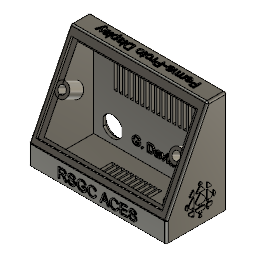
HalfSizeDisplayv4 (Autodesk Fusion 360 design; units mm, degrees)
Autodesk Fusion 360 part; units mm, degrees
sketch "Base" plane through (0, 0, 0) normal (0, 0, 1) x (1, 0, 0)
  line L0 (44.45, -19.685) -> (-44.45, -19.685)
  line L1 (-44.45, -19.685) -> (-44.45, 19.685)
  line L2 (-44.45, 19.685) -> (44.45, 19.685)
  line L3 (44.45, 19.685) -> (44.45, -19.685)
  line L4 (44.45, -19.685) -> (-44.45, 19.685) construction
  line L5 (-44.45, -19.685) -> (44.45, 19.685) construction
  line L6 (38.1, 15.875) -> (-38.1, 15.875)
  line L7 (-38.1, 15.875) -> (-38.1, -15.875)
  line L8 (-38.1, -15.875) -> (38.1, -15.875)
  line L9 (38.1, -15.875) -> (38.1, 15.875)
  line L10 (38.1, 15.875) -> (-38.1, -15.875) construction
  line L11 (-38.1, 15.875) -> (38.1, -15.875) construction
  dimension "d1" = 88.9
  dimension "d2" = 39.37
  dimension "d30" = 76.2
  dimension "d31" = 31.75
  constraint horizontal L0
  constraint perpendicular L0 L1
  constraint parallel L0 L2
  constraint parallel L1 L3
  constraint coincident L4 origin
  constraint coincident L5 origin
  constraint horizontal L6
  constraint perpendicular L6 L7
  constraint parallel L6 L8
  constraint parallel L7 L9
  constraint coincident L10 origin
  constraint coincident L11 origin
  measures "d1" distance of L1.end L2.end
  measures "d2" distance of L0.end L1.end
  measures "d30" distance of L7.end L8.end
  measures "d31" distance of L6.end L7.end
extrude "Extrude1" add sketch "Base" along normal blind 66.04 contours L0 L1 L2 L3 | L6 L7 L8 L9 makes body 1
sketch "2Points" plane through (44.45, 0, 0) normal (1, 0, 0) x (0, 1, 0)
  line L0 (-19.685, 0) -> (19.685, 0)
  line L1 (19.685, 0) -> (19.685, 66.04)
  line L2 (19.685, 66.04) -> (-19.685, 66.04)
  line L3 (-19.685, 66.04) -> (-19.685, 0)
  line L4 (6.9804, 66.04) -> (-19.685, 12.7041)
  point P0 (6.9804, 66.04)
  point P1 (-19.685, 12.7041)
  constraint coincident L2 P0
  constraint coincident L3 P1
  constraint coincident P0 L4.start
  constraint coincident P1 L4.end
sketch "BaseFill" plane through (0, 0, 0) normal (0, 0, -1) x (1, 0, 0)
  line L0 (-44.45, -19.685) -> (44.45, -19.685)
  line L1 (44.45, -19.685) -> (44.45, 19.685)
  line L2 (44.45, 19.685) -> (-44.45, 19.685)
  line L3 (-44.45, 19.685) -> (-44.45, -19.685)
  line L4 (-39.37, 14.605) -> (-39.37, -14.605)
  line L5 (-39.37, -14.605) -> (39.37, -14.605)
  line L6 (39.37, -14.605) -> (39.37, 14.605)
  line L7 (39.37, 14.605) -> (-39.37, 14.605)
  dimension "d5" = -5.08
extrude "Extrude3" cut sketch "2Points" against normal blind 101.6 contours L2 L3 L4 bodies 1
sketch "PermaProto" plane through (0, -20.83, 10.414) normal (0, -0.894444, 0.44718) x (1, 0, 0)
  line L0 (-44.45, 62.1906) -> (-44.45, 2.5604)
  line L1 (-44.45, 2.5604) -> (44.45, 2.5604)
  line L2 (44.45, 2.5604) -> (44.45, 62.1906)
  line L3 (44.45, 62.1906) -> (-44.45, 62.1906)
  line L4 (40.259, 57.023) -> (-41.275, 57.023)
  line L5 (-41.275, 57.023) -> (-41.275, 5.969)
  line L6 (-41.275, 5.969) -> (40.259, 5.969)
  line L7 (40.259, 5.969) -> (40.259, 57.023)
  line L8 (40.259, 57.023) -> (-41.275, 5.969) construction
  line L9 (-41.275, 57.023) -> (40.259, 5.969) construction
  point P0 (-0.508, 31.496)
  dimension "d25" = 81.534
  dimension "d26" = 51.054
  constraint horizontal L4
  constraint perpendicular L4 L5
  constraint parallel L4 L6
  constraint parallel L5 L7
  constraint coincident L8 P0
  constraint coincident L9 P0
  measures "d25" distance of L5.end L6.end
  measures "d26" distance of L4.end L5.end
extrude "Extrude6" cut sketch "PermaProto" against normal blind 1.5748 contours L4 L5 L6 L7 bodies 1
extrude "Extrude7" cut sketch "Base" along normal blind 59.69 contours L6 L7 L8 L9 bodies 1
fillet "Fillet5" radius 1.27 1 edges at (44.45, -19.685, 6.3521) on bodies 1
fillet "Fillet6" radius 1.27 1 edges at (-44.45, -19.685, 6.3521) on bodies 1
sketch "RSGC ACES" plane through (0, -19.685, 0) normal (0, -1, 0) x (1, 0, 0)
  line L0 (-43.18, 12.7041) -> (-43.18, 0)
  line L1 (-43.18, 0) -> (43.18, 0)
  line L2 (43.18, 0) -> (43.18, 12.7041)
  line L3 (43.18, 12.7041) -> (-43.18, 12.7041)
  line L4 (-35.052, 1.524) -> (35.56, 1.524) construction
  line L5 (35.56, 1.524) -> (35.56, 10.16) construction
  line L6 (35.56, 10.16) -> (-35.052, 10.16) construction
  line L7 (-35.052, 10.16) -> (-35.052, 1.524) construction
  dimension "d38" = 6.35
  text T0 "RSGC ACES" font "Arial" height 6.35 align centre middle in box 70.612 x 8.636 at (-35.052, 1.524) x (1, 0) y (0, 1) spacing 1 kerned
extrude "Extrude8" add sketch "RSGC ACES" along normal blind 0.508 text T0 bodies 1
fillet "Fillet7" radius 1.27 1 edges at (44.45, 19.685, 33.02) on bodies 1
fillet "Fillet8" radius 1.27 1 edges at (-44.45, 19.685, 33.02) on bodies 1
sketch "TopText" plane through (0, 0, 66.04) normal (0, 0, 1) x (-1, 0, 0)
  arc A0 (43.18, -19.685) -> (44.45, -18.415) centre (43.18, -18.415) ccw
  line L0 (44.45, -18.415) -> (44.45, -6.9804)
  line L1 (44.45, -6.9804) -> (-44.45, -6.9804)
  line L2 (-44.45, -6.9804) -> (-44.45, -18.415)
  arc A1 (-44.45, -18.415) -> (-43.18, -19.685) centre (-43.18, -18.415) ccw
  line L3 (-43.18, -19.685) -> (43.18, -19.685)
  line L4 (-44.2048, -20.7361) -> (45.0445, -20.5016) construction
  line L5 (45.0445, -20.5016) -> (45.0031, -4.76) construction
  line L6 (45.0031, -4.76) -> (-44.2462, -4.9945) construction
  line L7 (-44.2462, -4.9945) -> (-44.2048, -20.7361) construction
  dimension "d45" = 5.08
  text T0 "Perma-Proto Display" font "Arial" height 5.08 align centre middle in box 89.2496 x 15.7417 at (-44.2048, -20.7361) x (0.999997, 0.002627) y (-0.002627, 0.999997) spacing 1 kerned
extrude "Extrude9" add sketch "TopText" along normal blind 0.508 text T0 bodies 1
fillet "Fillet9" radius 1.27 5 edges at (44.45, -5.7173, 40.6422) (44.078, -19.313, 13.4481) (0, -19.685, 12.7041) (-44.078, -19.313, 13.4481) (-44.45, -5.7173, 40.6422) on bodies 1
fillet "Fillet10" radius 1.27 8 edges at (44.078, 7.3963, 66.04) (44.45, 13.4077, 66.04) (44.078, 19.313, 66.04) (0, 19.685, 66.04) (-44.078, 19.313, 66.04) (-44.45, 13.4077, 66.04) (-44.078, 7.3963, 66.04) (0, 6.9804, 66.04) on bodies 1
sketch "Revised_ACESLogoOutline-01" plane through (44.45, 0, 0) normal (1, 0, 0) x (0, 1, 0)
  arc A0 (1.4641, 12.3032) -> (0.4552, 12.1444) centre (0.401, 15.7741) cw
  spline S0 degree 3 poles (0.4552, 12.1444) (-0.3472, 12.1908) (-1.0048, 12.7982) (-1.1147, 13.5944) knots 1 1 1 1 2 2 2 2
  arc A1 (-1.1147, 13.5944) -> (-0.6596, 14.9843) centre (0.7846, 13.742) cw
  spline S1 degree 3 poles (-0.6596, 14.9843) (0.0742, 15.8839) (0.8185, 16.7764) (1.5523, 17.6795) knots 3 3 3 3 4 4 4 4
  spline S2 degree 3 poles (1.5523, 17.6795) (1.7123, 17.8877) (2.0105, 17.9271) (2.219, 17.7677) knots 4 4 4 4 5 5 5 5
  arc A2 (2.219, 17.7677) -> (2.3072, 17.6795) centre (1.9721, 17.4326) cw
  spline S3 degree 3 poles (2.3072, 17.6795) (2.7482, 17.1186) (3.2174, 16.5859) (3.669, 16.0356) knots 6 6 6 6 7 7 7 7
  arc A3 (3.669, 16.0356) -> (4.685, 14.7726) centre (-6.6786, 6.6712) cw
  spline S4 degree 3 poles (4.685, 14.7726) (5.2142, 14.0329) (5.0455, 13.0043) (4.3075, 12.4725) knots 8 8 8 8 9 9 9 9
  arc A4 (4.3075, 12.4725) -> (3.7219, 12.2079) centre (3.3301, 13.8553) cw
  arc A5 (3.7219, 12.2079) -> (2.5895, 12.2644) centre (3.2701, 14.5316) cw
  spline S5 degree 3 poles (2.5895, 12.2644) (2.526, 12.2644) (2.4413, 12.3455) (2.3566, 12.2397) (2.4237, 12.1656) (2.4448, 12.1021) knots 11 11 11 11 12 12 13 13 13 13
  arc A6 (2.4448, 12.1021) -> (2.8082, 11.4565) centre (6.0267, 13.6931) ccw
  spline S6 degree 3 poles (2.8082, 11.4565) (2.854, 11.386) (2.914, 11.3119) (2.8082, 11.1284) (2.72, 11.1461) (2.6318, 11.1461) knots 14 14 14 14 15 15 16 16 16 16
  line L0 (2.6318, 11.1461) -> (1.2207, 11.1461)
  arc A7 (1.2207, 11.1461) -> (1.0408, 11.2272) centre (1.2028, 11.3464) cw
  spline S7 degree 3 poles (1.0408, 11.2272) (0.9914, 11.3013) (1.0408, 11.3613) (1.069, 11.4213) knots 18 18 18 18 19 19 19 19
  arc A8 (1.069, 11.4213) -> (1.4641, 12.3032) centre (-1.2514, 12.9903) ccw
  arc A9 (2.3813, 8.1581) -> (2.7694, 7.3008) centre (5.1756, 8.9065) ccw
  arc A10 (2.7694, 7.3008) -> (2.8364, 7.202) centre (2.0017, 6.7077) cw
  spline S8 degree 3 poles (2.8364, 7.202) (2.8778, 7.1337) (2.856, 7.0448) (2.7876, 7.0034) knots 2 2 2 2 3 3 3 3
  spline S9 degree 3 poles (2.7876, 7.0034) (2.7863, 7.0025) (2.7849, 7.0017) (2.7835, 7.0009) knots 3 3 3 3 4 4 4 4
  arc A11 (2.7835, 7.0009) -> (2.6988, 6.9798) centre (2.7131, 7.1024) cw
  line L1 (2.6988, 6.9798) -> (1.1501, 6.9798)
  spline S10 degree 3 poles (1.1501, 6.9798) (1.0055, 6.9798) (0.949, 7.0927) (1.0267, 7.2197) knots 6 6 6 6 7 7 7 7
  arc A12 (1.0267, 7.2197) -> (1.4218, 7.9923) centre (-2.0573, 9.2842) ccw
  spline S11 degree 3 poles (1.4218, 7.9923) (1.4394, 8.0416) (1.4712, 8.0981) (1.3724, 8.1686) (1.3406, 8.1334) (1.2983, 8.1122) knots 8 8 8 8 9 9 10 10 10 10
  arc A13 (1.2983, 8.1122) -> (-0.134, 8.1334) centre (0.6138, 10.2674) cw
  spline S12 degree 3 poles (-0.134, 8.1334) (-0.7278, 8.3877) (-1.1181, 8.9657) (-1.1323, 9.6115) knots 11 11 11 11 12 12 12 12
  arc A14 (-1.1323, 9.6115) -> (-1.0724, 10.0983) centre (0.7514, 9.6266) cw
  spline S13 degree 3 poles (-1.0724, 10.0983) (-1.058, 10.1805) (-0.9825, 10.2375) (-0.8995, 10.2289) knots 13 13 13 13 14 14 14 14
  line L2 (-0.8995, 10.2289) -> (4.6638, 10.2289)
  spline S14 degree 3 poles (4.6638, 10.2289) (4.8225, 10.2289) (4.8931, 10.1759) (4.9248, 10.0313) knots 15 15 15 15 16 16 16 16
  spline S15 degree 3 poles (4.9248, 10.0313) (5.1442, 9.1603) (4.6159, 8.2764) (3.7449, 8.0571) knots 16 16 16 16 17 17 17 17
  line L3 (3.7449, 8.0571) -> (3.7395, 8.0558)
  line L4 (3.7395, 8.0558) -> (3.6866, 8.0558)
  arc A15 (3.6866, 8.0558) -> (2.3813, 8.1581) centre (3.238, 10.7098) cw
  spline S16 degree 3 poles (-2.9668, 12.3032) (-3.1961, 12.2468) (-3.4148, 12.2009) (-3.6335, 12.1656) knots 0 0 0 0 1 1 1 1
  spline S17 degree 3 poles (-3.6335, 12.1656) (-4.5393, 12.0182) (-5.393, 12.633) (-5.5405, 13.5387) (-5.618, 14.0149) (-5.4847, 14.5013) (-5.1752, 14.8714) knots 1 1 1 1 2 2 2 3 3 3 3
  spline S18 degree 3 poles (-5.1752, 14.8714) (-4.7413, 15.4323) (-4.2791, 15.9686) (-3.8346, 16.5154) knots 3 3 3 3 4 4 4 4
  line L5 (-3.8346, 16.5154) -> (-2.8751, 17.6866)
  arc A16 (-2.8751, 17.6866) -> (-2.5223, 17.863) centre (-2.5329, 17.4433) cw
  spline S19 degree 3 poles (-2.5223, 17.863) (-2.4347, 17.867) (-2.3605, 17.7992) (-2.3565, 17.7116) knots 6 6 6 6 7 7 7 7
  line L6 (-2.3565, 17.7116) -> (-2.3565, 17.7113)
  line L7 (-2.3565, 17.7113) -> (-2.3565, 11.3048)
  spline S20 degree 3 poles (-2.3565, 11.3048) (-2.3367, 11.2144) (-2.3933, 11.1248) (-2.4835, 11.1038) knots 9 9 9 9 10 10 10 10
  line L8 (-2.4835, 11.1038) -> (-3.2384, 11.1038)
  arc A17 (-3.2384, 11.1038) -> (-3.4289, 11.199) centre (-3.263, 11.2927) cw
  spline S21 degree 3 poles (-3.4289, 11.199) (-3.4748, 11.266) (-3.4289, 11.3225) (-3.3937, 11.3754) knots 12 12 12 12 13 13 13 13
  arc A18 (-3.3937, 11.3754) -> (-2.9668, 12.3032) centre (-5.9686, 13.1222) ccw
  line L9 (6.2195, 14.4975) -> (6.2195, 17.5984)
  spline S22 degree 3 poles (6.2195, 17.5984) (6.2195, 17.6901) (6.1807, 17.8065) (6.3007, 17.8489) knots 1 1 1 1 2 2 2 2
  arc A19 (6.3007, 17.8489) -> (6.6252, 17.7783) centre (6.402, 17.5331) cw
  arc A20 (6.6252, 17.7783) -> (6.9498, 17.4008) centre (4.8654, 15.9369) cw
  spline S23 degree 3 poles (6.9498, 17.4008) (7.6377, 16.5718) (8.3362, 15.7463) (9.003, 14.8996) knots 4 4 4 4 5 5 5 5
  spline S24 degree 3 poles (9.003, 14.8996) (9.6101, 14.2116) (9.5446, 13.1616) (8.8565, 12.5544) (8.4802, 12.2222) (7.9738, 12.0781) (7.479, 12.1621) knots 5 5 5 5 6 6 6 7 7 7 7
  spline S25 degree 3 poles (7.479, 12.1621) (7.2885, 12.1903) (7.105, 12.2221) (6.918, 12.2679) knots 7 7 7 7 8 8 8 8
  spline S26 degree 3 poles (6.918, 12.2679) (6.8898, 12.2679) (6.8651, 12.3067) (6.8087, 12.2291) (6.8369, 12.215) (6.8369, 12.1833) knots 8 8 8 8 9 9 10 10 10 10
  arc A21 (6.8369, 12.1833) -> (7.165, 11.4777) centre (9.9613, 13.2071) ccw
  spline S27 degree 3 poles (7.165, 11.4777) (7.2214, 11.3789) (7.3343, 11.2872) (7.2003, 11.0403) (7.0592, 11.0932) (6.9498, 11.0896) knots 11 11 11 11 12 12 13 13 13 13
  line L10 (6.9498, 11.0896) -> (6.4206, 11.0896)
  spline S28 degree 3 poles (6.4206, 11.0896) (6.2442, 11.0896) (6.216, 11.1249) (6.216, 11.2907) knots 14 14 14 14 15 15 15 15
  line L11 (6.216, 11.2907) -> (6.2195, 14.4975)
  line L12 (4.3216, 18.7943) -> (2.9916, 18.7943)
  spline S29 degree 3 poles (2.9916, 18.7943) (2.4872, 18.7943) (1.9792, 18.7696) (1.4747, 18.7943) knots 1 1 1 1 2 2 2 2
  line L13 (1.4747, 18.7943) -> (-0.5855, 18.7943)
  arc A22 (-0.5855, 18.7943) -> (-0.7584, 18.8825) centre (-0.6031, 18.9734) cw
  ellipse E0 centre (-0.6239, 18.9476) end of major axis (-0.5922, 19.0947) minor radius 0.1488 (-0.7196, 19.0624) -> (-0.7584, 18.8825) ccw
  arc A23 (-0.7196, 19.0624) -> (1.5523, 21.8211) centre (496.7599, -388.3118) cw
  spline S30 degree 3 poles (1.5523, 21.8211) (1.69, 22.0282) (1.9691, 22.0849) (2.1767, 21.9481) knots 6 6 6 6 7 7 7 7
  arc A24 (2.1767, 21.9481) -> (2.3178, 21.8) centre (1.9393, 21.5807) cw
  spline S31 degree 3 poles (2.3178, 21.8) (2.6318, 21.4084) (2.9599, 21.0274) (3.2809, 20.6393) knots 8 8 8 8 9 9 9 9
  line L14 (3.2809, 20.6393) -> (4.3392, 19.3446)
  spline S32 degree 3 poles (4.3392, 19.3446) (4.4168, 19.2494) (4.4909, 19.1541) (4.5721, 19.0659) knots 10 10 10 10 11 11 11 11
  ellipse E1 centre (4.4795, 18.9531) end of major axis (4.4479, 19.0966) minor radius 0.1453 (4.6109, 18.8896) -> (4.5721, 19.0659) ccw
  spline S33 degree 3 poles (4.6109, 18.8896) (4.5836, 18.8225) (4.5126, 18.7841) (4.4415, 18.7978) knots 12 12 12 12 13 13 13 13
  arc A25 (4.4415, 18.7978) -> (4.3216, 18.7943) centre (4.3918, 18.4486) ccw
  arc A26 (6.8616, 8.151) -> (7.2673, 7.2902) centre (9.9331, 9.0726) ccw
  spline S34 degree 3 poles (7.2673, 7.2902) (7.3096, 7.2232) (7.359, 7.1597) (7.2673, 6.9833) (7.1862, 7.0045) (7.1156, 7.0045) knots 1 1 1 1 2 2 3 3 3 3
  line L15 (7.1156, 7.0045) -> (6.4383, 7.0045)
  spline S35 degree 3 poles (6.4383, 7.0045) (6.3042, 7.0045) (6.2513, 7.0609) (6.2513, 7.195) knots 4 4 4 4 5 5 5 5
  line L16 (6.2513, 7.195) -> (6.2513, 10.0454)
  spline S36 degree 3 poles (6.2513, 10.0454) (6.2513, 10.1759) (6.3077, 10.243) (6.4383, 10.243) knots 6 6 6 6 7 7 7 7
  line L17 (6.4383, 10.243) -> (9.204, 10.243)
  spline S37 degree 3 poles (9.204, 10.243) (9.2869, 10.2543) (9.3647, 10.2009) (9.384, 10.1195) knots 8 8 8 8 9 9 9 9
  spline S38 degree 3 poles (9.384, 10.1195) (9.6305, 9.2477) (9.1236, 8.3411) (8.2518, 8.0946) knots 9 9 9 9 10 10 10 10
  line L18 (8.2518, 8.0946) -> (8.2515, 8.0946)
  arc A27 (8.2515, 8.0946) -> (8.0222, 8.0487) centre (7.7917, 9.7975) cw
  arc A28 (8.0222, 8.0487) -> (6.9639, 8.1686) centre (7.8052, 10.8626) cw
  line L19 (6.9639, 8.1686) -> (6.9039, 8.1686)
  line L20 (6.9039, 8.1686) -> (6.8616, 8.151)
  arc A29 (-2.9703, 8.1545) -> (-3.9581, 8.0099) centre (-4.0006, 11.7456) cw
  spline S39 degree 3 poles (-3.9581, 8.0099) (-4.5465, 8.018) (-5.0852, 8.3412) (-5.3692, 8.8566) knots 1 1 1 1 2 2 2 2
  arc A30 (-5.3692, 8.8566) -> (-5.5138, 10.0454) centre (-4.0161, 9.6244) cw
  spline S40 degree 3 poles (-5.5138, 10.0454) (-5.4945, 10.1433) (-5.4052, 10.2114) (-5.3057, 10.2042) knots 3 3 3 3 4 4 4 4
  line L21 (-5.3057, 10.2042) -> (-2.5858, 10.2042)
  spline S41 degree 3 poles (-2.5858, 10.2042) (-2.4059, 10.2042) (-2.3741, 10.1654) (-2.3741, 9.9784) knots 5 5 5 5 6 6 6 6
  line L22 (-2.3741, 9.9784) -> (-2.3741, 7.1879)
  spline S42 degree 3 poles (-2.3741, 7.1879) (-2.3741, 7.0362) (-2.4235, 6.9798) (-2.5787, 6.9798) knots 7 7 7 7 8 8 8 8
  line L23 (-2.5787, 6.9798) -> (-3.2314, 6.9798)
  arc A31 (-3.2314, 6.9798) -> (-3.4289, 7.0609) centre (-3.267, 7.1741) cw
  spline S43 degree 3 poles (-3.4289, 7.0609) (-3.4783, 7.1421) (-3.4289, 7.195) (-3.3901, 7.2549) knots 10 10 10 10 11 11 11 11
  arc A32 (-3.3901, 7.2549) -> (-2.9703, 8.1545) centre (-5.8179, 8.9356) ccw
  line L24 (6.2478, 20.3889) -> (6.2478, 21.8)
  spline S44 degree 3 poles (6.2478, 21.8) (6.2478, 21.9869) (6.336, 22.0646) (6.5441, 22.0046) knots 1 1 1 1 2 2 2 2
  arc A33 (6.5441, 22.0046) -> (6.7522, 21.8635) centre (6.4213, 21.5994) cw
  line L25 (6.7522, 21.8635) -> (7.8106, 20.5653)
  line L26 (7.8106, 20.5653) -> (8.9888, 19.1541)
  arc A34 (8.9888, 19.1541) -> (9.0806, 19.0342) centre (8.5621, 18.7328) cw
  spline S45 degree 3 poles (9.0806, 19.0342) (9.12, 18.9738) (9.103, 18.893) (9.0427, 18.8535) knots 6 6 6 6 7 7 7 7
  ellipse E2 centre (8.9485, 18.9568) end of major axis (9.0919, 18.9206) minor radius 0.1252 (9.0382, 18.8508) -> (9.0427, 18.8535) ccw
  arc A35 (9.0382, 18.8508) -> (8.9642, 18.8296) centre (8.9619, 18.9777) cw
  line L27 (8.9642, 18.8296) -> (6.3818, 18.8296)
  spline S46 degree 3 poles (6.3818, 18.8296) (6.2548, 18.8296) (6.2442, 18.9178) (6.2442, 19.0166) knots 10 10 10 10 11 11 11 11
  line L28 (6.2442, 19.0166) -> (6.2442, 20.3889)
  line L29 (6.2442, 20.3889) -> (6.2478, 20.3889)
  spline S47 degree 3 poles (-2.3847, 20.7487) (-2.353, 20.3465) (-2.4023, 19.8703) (-2.3635, 19.3976) knots 0 0 0 0 1 1 1 1
  line L30 (-2.3635, 19.3976) -> (-2.3635, 18.9495)
  spline S48 degree 3 poles (-2.3635, 18.9495) (-2.3575, 18.866) (-2.4204, 18.7933) (-2.5039, 18.7873) knots 2 2 2 2 3 3 3 3
  line L31 (-2.5039, 18.7873) -> (-2.5047, 18.7873)
  line L32 (-2.5047, 18.7873) -> (-4.1133, 18.7873)
  line L33 (-4.1133, 18.7873) -> (-5.0658, 18.7873)
  spline S49 degree 3 poles (-5.0658, 18.7873) (-5.1414, 18.7791) (-5.2092, 18.8337) (-5.2174, 18.9093) knots 6 6 6 6 7 7 7 7
  line L34 (-5.2174, 18.9093) -> (-5.2175, 18.9107)
  arc A36 (-5.2175, 18.9107) -> (-5.1717, 19.0271) centre (-5.0732, 18.9211) cw
  spline S50 degree 3 poles (-5.1717, 19.0271) (-4.8189, 19.454) (-4.4661, 19.8809) (-4.1133, 20.3007) knots 9 9 9 9 10 10 10 10
  line L35 (-4.1133, 20.3007) -> (-3.189, 21.4895)
  spline S51 degree 3 poles (-3.189, 21.4895) (-3.0867, 21.6165) (-2.9809, 21.7471) (-2.8751, 21.8705) knots 11 11 11 11 12 12 12 12
  arc A37 (-2.8751, 21.8705) -> (-2.5717, 22.0116) centre (-2.5561, 21.5815) cw
  spline S52 degree 3 poles (-2.5717, 22.0116) (-2.4866, 22.0223) (-2.409, 21.9619) (-2.3984, 21.8769) (-2.3967, 21.863) (-2.3968, 21.849) (-2.3988, 21.8353) knots 13 13 13 13 14 14 14 15 15 15 15
  spline S53 degree 3 poles (-2.3988, 21.8353) (-2.3882, 21.4966) (-2.3847, 21.1579) (-2.3847, 20.7487) knots 15 15 15 15 16 16 16 16
  line L36 (10.2977, 13.9471) -> (10.2977, 15.4182)
  spline S54 degree 3 poles (10.2977, 15.4182) (10.2977, 15.4994) (10.2977, 15.577) (10.3858, 15.6087) knots 1 1 1 1 2 2 2 2
  spline S55 degree 3 poles (10.3858, 15.6087) (10.4537, 15.6406) (10.5346, 15.6181) (10.5763, 15.5558) knots 2 2 2 2 3 3 3 3
  spline S56 degree 3 poles (10.5763, 15.5558) (10.781, 15.2842) (11.0314, 15.0443) (11.2113, 14.7515) knots 3 3 3 3 4 4 4 4
  spline S57 degree 3 poles (11.2113, 14.7515) (11.6071, 14.1883) (11.6155, 13.4396) (11.2325, 12.8676) knots 4 4 4 4 5 5 5 5
  arc A38 (11.2325, 12.8676) -> (10.5693, 12.3103) centre (9.8008, 13.8979) cw
  spline S58 degree 3 poles (10.5693, 12.3103) (10.3929, 12.2185) (10.2906, 12.2891) (10.2906, 12.4902) knots 6 6 6 6 7 7 7 7
  line L37 (10.2906, 12.4902) -> (10.2906, 13.9471)
  line L38 (10.2906, 13.9471) -> (10.2977, 13.9471)
  line L39 (-6.4593, 13.926) -> (-6.4593, 12.4796)
  ellipse E3 centre (-7.7786, 14.3773) end of major axis (-9.0268, 16.4702) minor radius 0.4973 (-6.7274, 12.3103) -> (-6.4593, 12.4796) ccw
  spline S59 degree 3 poles (-6.7274, 12.3103) (-7.2045, 12.5304) (-7.5452, 12.9684) (-7.6411, 13.485) knots 2 2 2 2 3 3 3 3
  ellipse E4 centre (-5.9166, 13.7823) end of major axis (-5.4476, 15.475) minor radius 1.7485 (-7.2425, 14.9243) -> (-7.6411, 13.485) ccw
  spline S60 degree 3 poles (-7.2425, 14.9243) (-7.0696, 15.1395) (-6.9003, 15.3371) (-6.7168, 15.5629) knots 4 4 4 4 5 5 5 5
  ellipse E5 centre (-6.598, 15.4782) end of major axis (-6.4565, 15.5178) minor radius 0.1453 (-6.5404, 15.6123) -> (-6.7168, 15.5629) ccw
  spline S61 degree 3 poles (-6.5404, 15.6123) (-6.4628, 15.584) (-6.4452, 15.5241) (-6.4452, 15.4464) knots 6 6 6 6 7 7 7 7
  spline S62 degree 3 poles (-6.4452, 15.4464) (-6.4628, 14.942) (-6.4593, 14.441) (-6.4593, 13.926) knots 7 7 7 7 8 8 8 8
  line L40 (1.9157, 22.8795) -> (0.8573, 22.8795)
  spline S63 degree 3 poles (0.8573, 22.8795) (0.7762, 22.8795) (0.7056, 22.8795) (0.628, 23.0629) (0.6668, 23.1053) (0.7233, 23.1617) knots 1 1 1 1 2 2 3 3 3 3
  line L41 (0.7233, 23.1617) -> (1.584, 24.22)
  spline S64 degree 3 poles (1.584, 24.22) (1.7517, 24.4069) (2.039, 24.4226) (2.2261, 24.2553) knots 4 4 4 4 5 5 5 5
  ellipse E6 centre (2.0099, 24.004) end of major axis (2.3392, 23.9648) minor radius 0.3315 (2.2614, 24.22) -> (2.2261, 24.2553) ccw
  spline S65 degree 3 poles (2.2614, 24.22) (2.5612, 23.8673) (2.847, 23.5145) (3.1398, 23.1441) knots 6 6 6 6 7 7 7 7
  spline S66 degree 3 poles (3.1398, 23.1441) (3.1857, 23.0911) (3.235, 23.0382) (3.1892, 22.9571) knots 7 7 7 7 8 8 8 8
  ellipse E7 centre (3.032, 23.0468) end of major axis (3.1973, 23.1231) minor radius 0.1804 (2.9987, 22.8689) -> (3.1892, 22.9571) ccw
  line L42 (2.9987, 22.8689) -> (1.9157, 22.8795)
  line L43 (1.9333, 4.6338) -> (1.1607, 4.6338)
  arc A39 (1.1607, 4.6338) -> (1.0055, 4.7044) centre (1.135, 4.7833) cw
  arc A40 (1.0055, 4.7044) -> (1.0302, 4.8878) centre (1.1625, 4.7766) cw
  arc A41 (1.0302, 4.8878) -> (1.4606, 5.7839) centre (-1.2782, 6.548) ccw
  line L44 (1.4606, 5.7839) -> (1.4606, 5.8121)
  spline S67 degree 3 poles (1.4606, 5.8121) (1.5311, 6.1649) (1.5311, 6.1649) (1.8768, 6.1649) knots 5 5 5 5 6 6 6 6
  line L45 (1.8768, 6.1649) -> (2.1485, 6.1649)
  spline S68 degree 3 poles (2.1485, 6.1649) (2.236, 6.1799) (2.3194, 6.1217) (2.3355, 6.0343) knots 7 7 7 7 8 8 8 8
  ellipse E8 centre (2.2911, 6.0238) end of major axis (2.2911, 6.0695) minor radius 0.0456 (2.3355, 6.0132) -> (2.3355, 6.0343) ccw
  arc A42 (2.3355, 6.0132) -> (2.8082, 4.9196) centre (4.6613, 6.3696) ccw
  arc A43 (2.8082, 4.9196) -> (2.847, 4.6938) centre (2.6238, 4.7716) cw
  spline S69 degree 3 poles (2.847, 4.6938) (2.8152, 4.6197) (2.7306, 4.6338) (2.66, 4.6338) knots 11 11 11 11 12 12 12 12
  line L46 (2.66, 4.6338) -> (1.9333, 4.6338)
extrude "Extrude10" add sketch "Revised_ACESLogoOutline-01" along normal blind 0.508 contours A0 S0 A1 S1 S2 A2 S3 A3 S4 A4 A5 S5 A6 S6 L0 A7 S7 A8 | S16 S17 S18 L5 A16 S19 L7 S20 L8 A17 S21 A18 | L12 S29 L13 A22 E0 A23 S30 A24 S31 L14 S32 E1 S33 A25 | A29 S39 A30 S40 L21 S41 L22 S42 L23 A31 S43 A32 | S47 L30 S48 L32 L33 S49 A36 S50 L35 S51 A37 S52 S53 | L39 E3 S59 E4 S60 E5 S61 S62 | L40 S63 L41 S64 E6 S65 S66 E7 L42 bodies 1
extrude "Extrude11" add sketch "Revised_ACESLogoOutline-01" against normal blind 6.35 contours A9 A10 S8 S9 A11 L1 S10 A12 S11 A13 S12 A14 S13 L2 S14 S15 L3 L4 A15 | L43 A39 A40 A41 L44 S67 L45 S68 E8 A42 A43 S69 L46 bodies 1
extrude "Extrude12" add sketch "Revised_ACESLogoOutline-01" along normal blind 0.508 contours A9 A10 S8 S9 A11 L1 S10 A12 S11 A13 S12 A14 S13 L2 S14 S15 L3 L4 A15 | L9 S22 A19 A20 S23 S24 S25 S26 A21 S27 L10 S28 L11 | A26 S34 L15 S35 L16 S36 L17 S37 S38 A27 A28 L19 L20 | L24 S44 A33 L25 L26 A34 S45 E2 A35 L27 S46 L28 L29 | L36 S54 S55 S56 S57 A38 S58 L37 L38 | L43 A39 A40 A41 L44 S67 L45 S68 E8 A42 A43 S69 L46 bodies 1
sketch "SChurterPJ" plane through (0, 19.685, 0) normal (0, 1, 0) x (-1, 0, 0)
  line L0 (43.18, 64.77) -> (-43.18, 64.77)
  line L1 (-43.18, 64.77) -> (-43.18, 0)
  line L2 (-43.18, 0) -> (43.18, 0)
  line L3 (43.18, 0) -> (43.18, 64.77)
  circle A0 centre (25.9132, 12.8698) radius 8.05
  circle A1 centre (25.9132, 12.8698) radius 6.5
  line L4 (31.8382, 9.1795) -> (19.9882, 9.1795)
  line L5 (19.9882, 9.1795) -> (19.9882, 16.5602)
  line L6 (19.9882, 16.5602) -> (31.8382, 16.5602)
  line L7 (31.8382, 16.5602) -> (31.8382, 9.1795)
  line L8 (31.8382, 9.1795) -> (19.9882, 16.5602) construction
  line L9 (19.9882, 9.1795) -> (31.8382, 16.5602) construction
  point P0 (25.9132, 12.8698)
  point P1 (25.9132, 12.8698)
  dimension "d58" = 16.1
  dimension "d59" = 13
  dimension "d67" = 11.85
  constraint concentric A0 A1
  constraint coincident P1 P0
  constraint horizontal L4
  constraint perpendicular L4 L5
  constraint parallel L4 L6
  constraint parallel L5 L7
  constraint coincident L8 P1
  constraint coincident L9 P1
  measures "d58" diameter of A0
  measures "d59" diameter of A1
  measures "d67" distance of L5.end L6.end
extrude "Extrude15" cut sketch "SChurterPJ" against normal blind 2 contours A0 | A1 L6 L7 | A1 L4 L7 | A1 L5 L6 | A1 L4 L5 bodies 1
extrude "Extrude16" cut sketch "SChurterPJ" against normal blind 10 contours A1 L4 L5 L6 L7 bodies 1
extrude "Extrude17" cut sketch "SChurterPJ" against normal blind 10 contours A1 L4 bodies 1
extrude "Extrude18" cut sketch "SChurterPJ" against normal blind 10 contours A1 L6 bodies 1
extrude "Extrude19" cut sketch "SChurterPJ" against normal blind 2 contours A1 L7 | A1 L5 bodies 1
sketch "LeftPier" plane through (-38.1, 0, 0) normal (1, 0, 0) x (0, 1, 0)
  line L0 (5.5664, 59.69) -> (-15.875, 16.8032)
  line L1 (-15.875, 16.8032) -> (-15.875, 0)
  line L2 (-15.875, 0) -> (15.875, 0)
  line L3 (15.875, 0) -> (15.875, 59.69)
  line L4 (15.875, 59.69) -> (5.5664, 59.69)
sketch "Sketch15" plane through (0, 0, 0) normal (0, 0, -1) x (1, 0, 0)
  arc A0 (-44.45, -18.415) -> (-43.18, -19.685) centre (-43.18, -18.415) ccw
  line L0 (-43.18, -19.685) -> (43.18, -19.685)
  arc A1 (43.18, -19.685) -> (44.45, -18.415) centre (43.18, -18.415) ccw
  line L1 (44.45, -18.415) -> (44.45, 18.415)
  arc A2 (44.45, 18.415) -> (43.18, 19.685) centre (43.18, 18.415) ccw
  line L2 (43.18, 19.685) -> (-43.18, 19.685)
  arc A3 (-43.18, 19.685) -> (-44.45, 18.415) centre (-43.18, 18.415) ccw
  line L3 (-44.45, 18.415) -> (-44.45, -18.415)
  line L4 (-38.1, 15.875) -> (38.1, 15.875)
  line L5 (38.1, 15.875) -> (38.1, -15.875)
  line L6 (38.1, -15.875) -> (-38.1, -15.875)
  line L7 (-38.1, -15.875) -> (-38.1, 15.875)
extrude "Extrude20" add sketch "Sketch15" against normal blind 2 contours L4 L5 L6 L7 bodies 1
extrude "Extrude21" cut sketch "Sketch15" against normal blind 5 contours L4 L5 L6 L7 bodies 1
sketch "Proto Plane" plane through (0, -19.4214, 9.7098) normal (0, -0.894444, 0.44718) x (1, 0, 0)
  line L0 (38.1, 7.9305) -> (-38.1, 7.9305)
  line L1 (-38.1, 7.9305) -> (-38.1, 55.8785)
  line L2 (-38.1, 55.8785) -> (38.1, 55.8785)
  line L3 (38.1, 55.8785) -> (38.1, 7.9305)
  line L4 (40.259, 5.969) -> (40.259, 57.023)
  line L5 (40.259, 57.023) -> (-41.275, 57.023)
  line L6 (-41.275, 57.023) -> (-41.275, 5.969)
  line L7 (-41.275, 5.969) -> (40.259, 5.969)
  circle A0 centre (36.342, 31.9045) radius 2.5
  circle A1 centre (36.342, 31.9045) radius 4.5
  circle A2 centre (-37.358, 31.9045) radius 2.5
  circle A3 centre (-37.358, 31.9045) radius 4.5
  dimension "d83" = 5
  dimension "d84" = 9
  dimension "d85" = 5
  dimension "d86" = 9
  constraint concentric A0 A1
  constraint concentric A2 A3
  measures "d83" diameter of A0
  measures "d84" diameter of A1
  measures "d85" diameter of A2
  measures "d86" diameter of A3
extrude "Extrude22" add sketch "Proto Plane" against normal blind 10 separate body contours L3 A0 | L3 A0 | L1 A2 | L1 A2 makes body 2 at (38.8389, 0.7529, 35.1539) makes body 3 at (-34.8611, 0.7529, 35.1539)
extrude "Extrude23" add sketch "Proto Plane" against normal blind 10 contours L3 A0 A1 | L3 L4 A0 A1 | L1 L6 A2 A3 | L1 A2 A3 | L4 A1 | L6 A3 bodies 2 3
extrude "Extrude24" cut sketch "Proto Plane" against normal blind 7 contours L3 A0 | L3 A0 | L1 A2 | L1 A2 bodies 2 3
extrude "Extrude25" cut sketch "Proto Plane" against normal blind 7 contours L3 A0 | L1 A2 picked at (38.3401, 31.795) picked at (-39.0646, 31.4605) bodies 1
sketch "ShortBase" plane through (0, 0, 0) normal (0, 0, -1) x (1, 0, 0)
  line L0 (38.1, 15.875) -> (38.1, -15.875)
  line L1 (38.1, -15.875) -> (-38.1, -15.875)
  line L2 (-38.1, -15.875) -> (-38.1, 15.875)
  line L3 (-38.1, 15.875) -> (38.1, 15.875)
  arc A0 (-44.45, -18.415) -> (-43.18, -19.685) centre (-43.18, -18.415) ccw
  line L4 (-43.18, -19.685) -> (43.18, -19.685)
  arc A1 (43.18, -19.685) -> (44.45, -18.415) centre (43.18, -18.415) ccw
  line L5 (44.45, -18.415) -> (44.45, 18.415)
  arc A2 (44.45, 18.415) -> (43.18, 19.685) centre (43.18, 18.415) ccw
  line L6 (43.18, 19.685) -> (-43.18, 19.685)
  arc A3 (-43.18, 19.685) -> (-44.45, 18.415) centre (-43.18, 18.415) ccw
  line L7 (-44.45, 18.415) -> (-44.45, -18.415)
  line L8 (-38.1, 15.875) -> (38.1, 15.875)
  line L9 (38.1, 15.875) -> (38.1, -15.875)
  line L10 (38.1, -15.875) -> (-38.1, -15.875)
  line L11 (-38.1, -15.875) -> (-38.1, 15.875)
  constraint horizontal L8
  constraint vertical L9
  constraint horizontal L10
  constraint vertical L11
  constraint coincident L0.end L1.start
  constraint coincident L2.end L3.start
extrude "Extrude26" add sketch "ShortBase" against normal blind 3 contours L0 L1 L2 L3 L8 L9 L10 L11 bodies 1
sketch "SchurterPJ2" plane through (0, 0, 0) normal (0, 0, -1) x (1, 0, 0)
  circle A0 centre (26.6513, -5.1831) radius 8
  circle A1 centre (26.6513, -5.1831) radius 6.5
  line L0 (32.6772, -2.7461) -> (20.6254, -2.7461)
  line L1 (20.6254, -2.7461) -> (20.6254, -7.6201)
  line L2 (20.6254, -7.6201) -> (32.6772, -7.6201)
  line L3 (32.6772, -7.6201) -> (32.6772, -2.7461)
  line L4 (32.6772, -2.7461) -> (20.6254, -7.6201) construction
  line L5 (20.6254, -2.7461) -> (32.6772, -7.6201) construction
  point P0 (26.6513, -5.1831)
  dimension "d97" = 16
  dimension "d98" = 13
  constraint concentric A0 A1
  constraint horizontal L0
  constraint perpendicular L0 L1
  constraint parallel L0 L2
  constraint parallel L1 L3
  constraint coincident L4 P0
  constraint coincident L5 P0
  constraint coincident A1 L0.start
  constraint coincident P0 A0.centre
  measures "d97" diameter of A0
  measures "d98" diameter of A1
extrude "Extrude30" cut sketch "SchurterPJ2" against normal blind 2 bodies 1
extrude "Extrude31" cut sketch "SchurterPJ2" against normal blind 2 contours A1 L3 bodies 1
extrude "Extrude32" cut sketch "SchurterPJ2" against normal blind 2 contours A1 L1 bodies 1
extrude "Extrude33" cut sketch "SchurterPJ2" against normal blind 4 contours A1 L0 | L0 L1 L2 L3 | A1 L2 bodies 1
sketch "Davidge" plane through (0, 15.875, 0) normal (0, -1, 0) x (1, 0, 0)
  line L0 (-38.1, 3) -> (38.1, 3)
  line L1 (38.1, 3) -> (38.1, 59.69)
  line L2 (38.1, 59.69) -> (-38.1, 59.69)
  line L3 (-38.1, 59.69) -> (-38.1, 3)
  arc A0 (-19.9882, 15.5427) -> (-31.8382, 15.5427) centre (-25.9132, 12.8698) ccw
  line L4 (-19.9882, 15.5427) -> (-19.9882, 10.1969)
  arc A1 (-31.8382, 10.1969) -> (-19.9882, 10.1969) centre (-25.9132, 12.8698) ccw
  line L5 (-31.8382, 10.1969) -> (-31.8382, 15.5427)
  line L6 (-12.2805, 8.2828) -> (32.9791, 8.2828) construction
  line L7 (32.9791, 8.2828) -> (32.9791, 15.9541) construction
  line L8 (32.9791, 15.9541) -> (-12.2805, 15.9541) construction
  line L9 (-12.2805, 15.9541) -> (-12.2805, 8.2828) construction
  dimension "d116" = 5.08
  text T0 "G. Davidge" font "Arial" height 5.08 align left top in box 45.2596 x 7.6713 at (-12.2805, 8.2828) x (1, 0) y (0, 1) spacing 1 kerned
extrude "Extrude35" add sketch "Davidge" along normal blind 1 text T0 bodies 1
sketch "Sketch22" plane through (0, 19.685, 0) normal (0, 1, 0) x (-1, 0, 0)
  line L0 (43.18, 64.77) -> (-43.18, 64.77)
  line L1 (-43.18, 64.77) -> (-43.18, 0)
  line L2 (-43.18, 0) -> (43.18, 0)
  line L3 (43.18, 0) -> (43.18, 64.77)
  circle A0 centre (25.9132, 12.8698) radius 8.05
sketch "GrillLong" plane through (0, 19.685, 32.385) normal (0, 1, 0) x (-1, 0, 0)
  line L0 (-1.21, 26.5498) -> (-1.21, 1.5498)
  line L1 (0.79, 26.5498) -> (0.79, 1.5498)
  line L2 (2.2186, 26.5498) -> (2.2186, 1.5498)
  line L3 (4.2186, 26.5498) -> (4.2186, 1.5498)
  line L4 (5.6471, 26.5498) -> (5.6471, 1.5498)
  line L5 (7.6471, 26.5498) -> (7.6471, 1.5498)
  line L6 (9.0757, 26.5498) -> (9.0757, 1.5498)
  line L7 (12.5043, 26.5498) -> (12.5043, 1.5498)
  line L8 (15.9329, 26.5498) -> (15.9329, 1.5498)
  line L9 (19.3614, 26.5498) -> (19.3614, 1.5498)
  line L10 (22.79, 26.5498) -> (22.79, 1.5498)
  line L11 (11.0757, 26.5498) -> (11.0757, 1.5498)
  line L12 (14.5043, 26.5498) -> (14.5043, 1.5498)
  line L13 (17.9329, 26.5498) -> (17.9329, 1.5498)
  line L14 (21.3614, 26.5498) -> (21.3614, 1.5498)
  line L15 (24.79, 26.5498) -> (24.79, 1.5498)
  line L16 (-4.6386, 26.5498) -> (-4.6386, 1.5498)
  line L17 (-8.0671, 26.5498) -> (-8.0671, 1.5498)
  line L18 (-11.4957, 26.5498) -> (-11.4957, 1.5498)
  line L19 (-14.9243, 26.5498) -> (-14.9243, 1.5498)
  line L20 (-18.3529, 26.5498) -> (-18.3529, 1.5498)
  line L21 (-21.7814, 26.5498) -> (-21.7814, 1.5498)
  line L22 (-25.21, 26.5498) -> (-25.21, 1.5498)
  line L23 (-2.6386, 26.5498) -> (-2.6386, 1.5498)
  line L24 (-6.0671, 26.5498) -> (-6.0671, 1.5498)
  line L25 (-9.4957, 26.5498) -> (-9.4957, 1.5498)
  line L26 (-12.9243, 26.5498) -> (-12.9243, 1.5498)
  line L27 (-16.3529, 26.5498) -> (-16.3529, 1.5498)
  line L28 (-19.7814, 26.5498) -> (-19.7814, 1.5498)
  line L29 (-23.21, 26.5498) -> (-23.21, 1.5498)
  line L30 (24.79, 1.5498) -> (-25.21, 1.5498)
  line L31 (-25.21, 26.5498) -> (24.79, 26.5498)
  constraint perpendicular L22 L30
  constraint perpendicular L15 L31
extrude "Extrude36" cut sketch "GrillLong" against normal blind 5 contours L0 L1 L30 L31 | L16 L23 L30 L31 | L2 L3 L30 L31 | L17 L24 L30 L31 | L4 L5 L30 L31 | L18 L25 L30 L31 | L6 L11 L30 L31 | L19 L26 L30 L31 | L7 L12 L30 L31 | L20 L27 L30 L31 | L8 L13 L30 L31 | L21 L28 L30 L31 | L9 L14 L30 L31 | L22 L29 L30 L31 | L10 L15 L30 L31 bodies 1
sketch "Sketch24" plane through (0, 0, 0) normal (0, 0, -1) x (1, 0, 0)
  arc A0 (-44.45, -18.415) -> (-43.18, -19.685) centre (-43.18, -18.415) ccw
  line L0 (-43.18, -19.685) -> (43.18, -19.685)
  arc A1 (43.18, -19.685) -> (44.45, -18.415) centre (43.18, -18.415) ccw
  line L1 (44.45, -18.415) -> (44.45, 18.415)
  arc A2 (44.45, 18.415) -> (43.18, 19.685) centre (43.18, 18.415) ccw
  line L2 (43.18, 19.685) -> (-43.18, 19.685)
  arc A3 (-43.18, 19.685) -> (-44.45, 18.415) centre (-43.18, 18.415) ccw
  line L3 (-44.45, 18.415) -> (-44.45, -18.415)
  circle A4 centre (26.6513, -5.1831) radius 8
  line L4 (-1, 11.9725) -> (-1, -5.7925)
  line L5 (-4, 11.9725) -> (-4, -5.7925)
  line L6 (-7, 11.9725) -> (-7, -5.7925)
  line L7 (-10, 11.9725) -> (-10, -5.7925)
  line L8 (-13, 11.9725) -> (-13, -5.7925)
  line L9 (-16, 11.9725) -> (-16, -5.7925)
  line L10 (2, 11.9725) -> (2, -5.7925)
  line L11 (5, 11.9725) -> (5, -5.7925)
  line L12 (8, 11.9725) -> (8, -5.7925)
  line L13 (11, 11.9725) -> (11, -5.7925)
  line L14 (14, 11.9725) -> (14, -5.7925)
  line L15 (-14, 11.9725) -> (-14, -5.7925)
  line L16 (-11, 11.9725) -> (-11, -5.7925)
  line L17 (-8, 11.9725) -> (-8, -5.7925)
  line L18 (-5, 11.9725) -> (-5, -5.7925)
  line L19 (-2, 11.9725) -> (-2, -5.7925)
  line L20 (1, 11.9725) -> (1, -5.7925)
  line L21 (4, 11.9725) -> (4, -5.7925)
  line L22 (7, 11.9725) -> (7, -5.7925)
  line L23 (10, 11.9725) -> (10, -5.7925)
  line L24 (13, 11.9725) -> (13, -5.7925)
  line L25 (16, 11.9725) -> (16, -5.7925)
  line L26 (-16, 11.9725) -> (11, 11.9725)
  line L27 (-16, 11.9725) -> (16, 11.9725) construction
  line L28 (-16, -5.7925) -> (16, -5.7925)
  line L29 (11, 11.9725) -> (16, 11.9725)
  constraint perpendicular L13 L26
  constraint perpendicular L25 L27
  constraint perpendicular L25 L28
extrude "Extrude37" cut sketch "Sketch24" against normal blind 5 contours L4 L20 L26 L28 | L5 L19 L26 L28 | L10 L21 L26 L28 | L6 L18 L26 L28 | L11 L22 L26 L28 | L7 L17 L26 L28 | L12 L23 L26 L28 | L8 L16 L26 L28 | L13 L24 L28 L29 | L9 L15 L26 L28 | L14 L25 L28 L29 bodies 1
